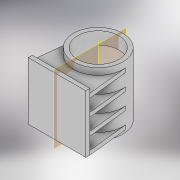
# Autodesk Inventor part: LENS MOUNT
Saved by Autodesk Inventor 2017 (Build 210142000, 142)
## iProperties
Created: 2017-04-01
Part Number: LENS MOUNT
Material: Generic
Document SubType Name: Modeling
Designer: Muchen
Density: 1 g/cm^3
Appearance: Default
Author: Muchen
Autodesk Inventor part; units mm, degrees
ref_plane "YZ Plane" through (0, 0, 0) normal (1, 0, 0) x (0, 1, 0)
ref_plane "XZ Plane" through (0, 0, 0) normal (0, 1, 0) x (-1, 0, 0)
ref_plane "XY Plane" through (0, 0, 0) normal (0, 0, 1) x (1, 0, 0)
sketch "Sketch1" plane through (0, 0, 0) normal (0, 1, 0) x (-1, 0, 0)
  line L0 (0, 0) -> (70, 0)
  line L1 (70, 0) -> (70, -70)
  line L2 (70, -70) -> (0, -70)
  line L3 (0, -70) -> (0, 0)
  dimension "d0" = 70
  dimension "d1" = 70
  constraints: 8 end point, 2 parallel, 1 horizontal, 1 perpendicular
  measures "d0" distance of L1.end L2.end
  measures "d1" distance of L2.end L0.start
extrude "Extrusion1" add sketch "Sketch1" along normal blind 5
ref_plane "Work Plane2" through (-70, 0, -35) normal (0, 0, 1) x (1, 0, 0)
sketch "Sketch2" plane through (-70, 0, -35) normal (0, 0, 1) x (1, 0, 0)
  circle A0 centre (35, 50) radius 25
  line L0 (35, 50) -> (35, 5) construction
  line L1 (70, 5) -> (0, 5)
  circle A1 centre (35, 50) radius 30
  line L2 (0, 5) -> (5.1712, 53.2002)
  line L3 (70, 5) -> (64.8288, 53.2002)
  point P0 (0, 0)
  dimension "d4" = 50
  dimension "d5" = 50
  dimension "d6" = 60
  constraints: 8 end point, 2 centre point, 2 point on circle, 2 tangent, 1 coincident, 1 midpoint, 1 vertical
  measures "d4" diameter of A0
  measures "d5" vertical distance of point (0, 0) L0.start
  measures "d6" diameter of A1
extrude "Extrusion2" add sketch "Sketch2" against normal blind 5 contours L1 L2 A1 L3
pattern_linear "Rectangular Pattern1" count 5 spacing 15 along (0, 0, -1) of "Extrusion2" first direction both ways yes
extrude "Extrusion3" add sketch "Sketch2" along normal mid plane 70 contours A1
ref_plane "Work Plane1" through (-35, 0, 0) normal (1, 0, 0) x (0, 0, -1)
sketch "Sketch3" plane through (-35, 0, 0) normal (1, 0, 0) x (0, 0, -1)
  line L0 (70, 75) -> (0, 75) projected
  line L1 (70, 80) -> (0, 80) projected
  line L2 (15, 75) -> (55, 75)
  line L3 (55, 75) -> (55, 80)
  line L4 (55, 80) -> (15, 80)
  line L5 (15, 80) -> (15, 75)
  line L6 (84, 50) -> (-14, 50) projected
  point P0 (0, 0)
  dimension "d19" = 15
  dimension "d20" = 15
  constraints: 8 end point, 2 parallel, 2 point on line, 1 horizontal, 1 perpendicular
  measures "d19" distance from line of L1.start L3
  measures "d20" distance from line of L1.end L5
revolve "Revolution1" cut sketch "Sketch3" angle 90 mid plane about axis through (-35, 50, -35) along (0, 0, 1)
body "Solid1"
